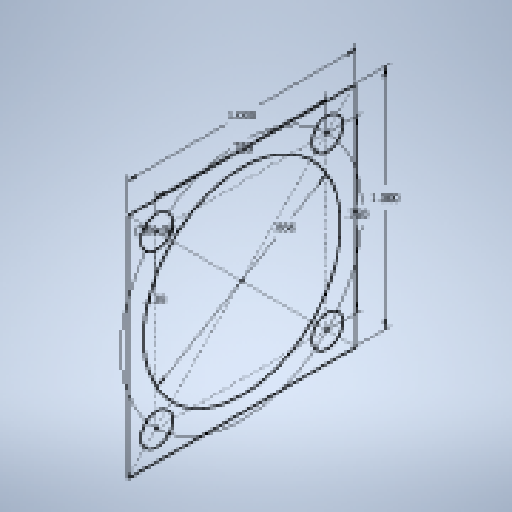
# Autodesk Inventor part: Motor Sleeve
Saved by Autodesk Inventor 2023.2 (Build 272271000, 271)
## iProperties
Created: 2022-12-29
Part Number: Motor Sleeve
Material: UHMW, Black
Document SubType Name: Modeling
Designer: Nathan Cai
Density: 0.94 g/cm^3
Appearance: Smooth - Black
Author: Nathan Cai
Autodesk Inventor part; units mm, degrees
ref_plane "YZ Plane" through (0, 0, 0) normal (1, 0, 0) x (0, 1, 0)
ref_plane "XZ Plane" through (0, 0, 0) normal (0, 1, 0) x (-1, 0, 0)
ref_plane "XY Plane" through (0, 0, 0) normal (0, 0, 1) x (1, 0, 0)
sketch "Sketch1" plane through (0, 0, 0) normal (1, 0, 0) x (0, 1, 0)
  circle A0 centre (0, 0) radius 11
  line L0 (-12.7, 12.7) -> (12.7, 12.7)
  line L1 (12.7, 12.7) -> (12.7, -12.7)
  line L2 (12.7, -12.7) -> (-12.7, -12.7)
  line L3 (-12.7, -12.7) -> (-12.7, 12.7)
  line L4 (-12.7, 12.7) -> (12.7, -12.7) construction
  line L5 (12.7, 12.7) -> (-12.7, -12.7) construction
  line L6 (-9.525, 9.525) -> (9.525, 9.525) construction
  line L7 (9.525, 9.525) -> (9.525, -9.525) construction
  line L8 (9.525, -9.525) -> (-9.525, -9.525) construction
  line L9 (-9.525, -9.525) -> (-9.525, 9.525) construction
  line L10 (-9.525, 9.525) -> (9.525, -9.525) construction
  line L11 (9.525, 9.525) -> (-9.525, -9.525) construction
  circle A1 centre (9.525, 9.525) radius 1.7526
  circle A2 centre (-9.525, 9.525) radius 1.7526
  circle A3 centre (-9.525, -9.525) radius 1.7526
  circle A4 centre (9.525, -9.525) radius 1.7526
  dimension "d0" = 22
  dimension "d1" = 25.4
  dimension "d2" = 25.4
  dimension "d3" = 19.05
  dimension "d4" = 19.05
  dimension "d5" = 3.5052
  dimension "d8" = 360
  constraints: 24 end point, 5 centre point, 4 midpoint, 4 parallel, 2 coincident, 2 horizontal, 2 perpendicular, 9 other
  measures "d0" diameter of A0
  measures "d1" distance of L1.end L2.end
  measures "d2" distance of L0.end L1.end
  measures "d3" distance of L7.end L8.end
  measures "d4" distance of L6.end L7.end
  measures "d5" diameter of A1
extrude "Extrusion1" add sketch "Sketch1" along normal blind 16.8
sketch "Sketch2" plane through (0, 12.7, 12.7) normal (0, 1, 0) x (1, 0, 0)
  circle A0 centre (13.625, -3.175) radius 3.175
  circle A1 centre (13.625, -3.175) radius 1.3891
  line L0 (0, 0) -> (16.8, 0) projected
  line L1 (16.8, 25.4) -> (16.8, 0) projected
  line L2 (0, 12.7) -> (16.8, 12.7) construction
  line L3 (11.3799, -5.4201) -> (5.9599, 0)
  line L4 (16.8, -3.175) -> (16.8, 0)
  circle A2 centre (13.625, 28.575) radius 3.175
  circle A3 centre (13.625, 28.575) radius 1.3891
  line L5 (0, 25.4) -> (16.8, 25.4)
  line L6 (11.3799, 30.8201) -> (5.9599, 25.4)
  line L7 (16.8, 28.575) -> (16.8, 25.4)
  dimension "d12" = 6.35
  dimension "d13" = 2.7781
  dimension "d14" = 45
  constraints: 12 end point, 6 symmetric about line, 4 centre point, 4 point on circle, 4 tangent, 2 coincident, 2 point on line, 1 midpoint, 1 perpendicular, 2 other
  measures "d12" diameter of A0
  measures "d13" diameter of A1
  measures "d14" angle of L4 L3
extrude "Extrusion2" add sketch "Sketch2" against normal up to surface (25.4 mm away)
fillet "Fillet1" radius 6.35 2 edges at (5.9599, 0, -12.7) (5.9599, 0, 12.7)
body "Solid1"
